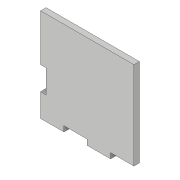
# Autodesk Inventor part: side2+hinge
Saved by Autodesk Inventor 2017 (Build 210142000, 142)
## iProperties
Created: 2019-05-21
Part Number: side2+hinge
Material: Generic
Document SubType Name: Modeling
Designer: markg
Density: 1 g/cm^3
Appearance: Default
Author: markg
Autodesk Inventor part; units mm, degrees
ref_plane "YZ Plane" through (0, 0, 0) normal (1, 0, 0) x (0, 1, 0)
ref_plane "XZ Plane" through (0, 0, 0) normal (0, 1, 0) x (-1, 0, 0)
ref_plane "XY Plane" through (0, 0, 0) normal (0, 0, 1) x (1, 0, 0)
sketch "Sketch1" plane through (0, 0, 0) normal (0, 0, 1) x (1, 0, 0)
  line L0 (-25.4, -25.4) -> (25.4, -25.4)
  line L1 (25.4, -25.4) -> (25.4, 25.4)
  line L2 (25.4, 25.4) -> (-25.4, 25.4)
  line L3 (-25.4, 25.4) -> (-25.4, -25.4)
  line L4 (-25.4, -25.4) -> (25.4, 25.4) construction
  line L5 (25.4, -25.4) -> (-25.4, 25.4) construction
  point P0 (0, 0)
  dimension "d0" = 50.8
  dimension "d1" = 50.8
  constraints: 12 end point, 2 midpoint, 2 parallel, 1 horizontal, 1 perpendicular
  measures "d0" distance of L2.end L1.end
  measures "d1" distance of L1.end L0.end
extrude "Extrusion1" add sketch "Sketch1" along normal blind 2.9718
sketch "Sketch2" plane through (0, 0, 2.9718) normal (0, 0, 1) x (1, 0, 0)
  line L0 (-25.4, -25.4) -> (25.4, -25.4) projected
  line L1 (25.4, -25.4) -> (12.7, -25.4)
  line L2 (12.7, -25.4) -> (12.7, -22.4282)
  line L3 (12.7, -22.4282) -> (25.4, -22.4282)
  line L4 (25.4, -22.4282) -> (25.4, -25.4)
  line L5 (0, -25.4) -> (-12.7, -25.4)
  line L6 (-12.7, -25.4) -> (-12.7, -22.4282)
  line L7 (-12.7, -22.4282) -> (0, -22.4282)
  line L8 (0, -22.4282) -> (0, -25.4)
  line L9 (-25.4, -12.7) -> (-22.4282, -12.7)
  line L10 (-22.4282, -12.7) -> (-22.4282, 0)
  line L11 (-22.4282, 0) -> (-25.4, 0)
  line L12 (-25.4, 0) -> (-25.4, -12.7)
  point P0 (0, 0)
  dimension "d4" = 12.7
  dimension "d5" = 2.9718
  dimension "d6" = 12.7
  dimension "d7" = 2.9718
  dimension "d8" = 2.9718
  dimension "d9" = 12.7
  dimension "d10" = 12.7
  constraints: 24 end point, 6 parallel, 3 horizontal, 3 perpendicular, 1 midpoint
  measures "d4" distance of L2.end L3.end
  measures "d5" distance of L1.end L2.end
  measures "d6" distance of L6.end L7.end
  measures "d7" distance of L5.end L6.end
  measures "d8" distance of L11.end L10.end
  measures "d9" distance of L10.end L9.end
  measures "d10" distance between parallel lines of L0 L9
extrude "Extrusion2" cut sketch "Sketch2" against normal blind 2.9718
body "Solid1"
